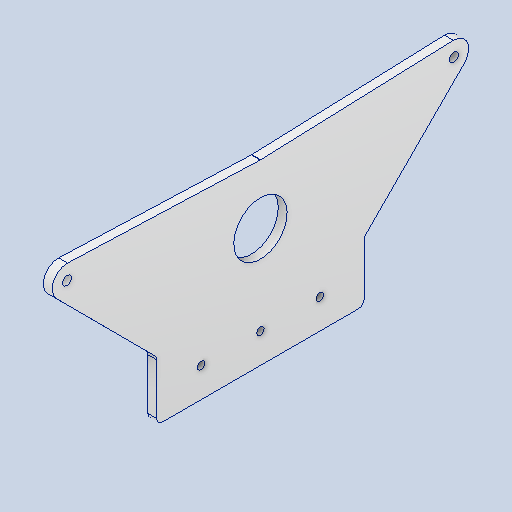
# Autodesk Inventor part: base_weel-v3-Plate-1
Saved by Autodesk Inventor 2025.2 (Build 292293000, 293)
## iProperties
Created: 2025-03-31
Part Number: base_weel-v3-Plate-1
Material: アルミニウム 6061
Document SubType Name: Modeling
Designer: haruy
Density: 2.7 g/cm^3
Appearance: アルミニウム - フラット
Author: haruy
Autodesk Inventor part; units mm, degrees
ref_plane "YZ Plane" through (0, 0, 0) normal (1, 0, 0) x (0, 1, 0)
ref_plane "XZ Plane" through (0, 0, 0) normal (0, 1, 0) x (-1, 0, 0)
ref_plane "XY Plane" through (0, 0, 0) normal (0, 0, 1) x (1, 0, 0)
sketch "スケッチ1" plane through (0, 0, 0) normal (1, 0, 0) x (0, 1, 0)
  line L0 (0, 0) -> (20, 0)
  line L1 (20, 0) -> (20, -110)
  line L2 (20, -110) -> (0, -110)
  line L3 (0, -110) -> (0, 0)
  circle A0 centre (40, -55) radius 52.5
  line L4 (-12.5, 72.5213) -> (-12.5, -343.3137)
  circle A1 centre (40, -55) radius 9.5 construction
  circle A2 centre (40, -55) radius 20
  circle A3 centre (68.2843, -26.7157) radius 20
  circle A4 centre (68.2843, -83.2843) radius 20
  line L5 (68.2843, -26.7157) -> (40, -55)
  line L6 (40, -55) -> (68.2843, -83.2843)
  line L7 (40, -55) -> (40, -2.5)
  line L8 (0, 15) -> (20, 15)
  line L9 (20, 15) -> (20, -125)
  line L10 (20, -125) -> (0, -125)
  line L11 (0, -125) -> (0, 15)
  circle A5 centre (68.2843, -26.7157) radius 23.5
  circle A6 centre (57.4091, 10.2164) radius 5
  circle A7 centre (57.4091, -120.2164) radius 5
  line L12 (20, -20) -> (0, -20)
  line L13 (0, -55) -> (20, -55)
  circle A8 centre (40, -55) radius 9
  circle A9 centre (57.4091, 10.2164) radius 1.5
  circle A10 centre (57.4091, -120.2164) radius 1.5
  line L14 (20, -20) -> (53.8799, 13.7583)
  line L15 (62.4057, 10.0326) -> (59.9865, -55.7352)
  circle A11 centre (10, -55) radius 1.25
  circle A12 centre (10, -35) radius 1.25
  line L16 (20, -90) -> (53.8799, -123.7583)
  line L17 (62.4057, -120.0326) -> (59.9865, -54.2648)
  circle A13 centre (10, -75) radius 1.25
  line L18 (20, -90) -> (0, -90)
  point P0 (0.8688, -20)
  point P1 (0, -20.9963)
  point P2 (0, -89.0037)
  point P3 (0.8688, -90)
  point P4 (60.0135, -55)
  point P5 (0, -90)
  point P6 (0, -20)
  dimension "d2" = 105
  dimension "d6" = 40
  dimension "d0" = 20
  dimension "d1" = 110
  dimension "d3" = 19
  dimension "d4" = 20
  dimension "d5" = 55
  dimension "d7" = 40
  dimension "d8" = 40
  dimension "d9" = 90
  dimension "d10" = 45
  dimension "d11" = 20
  dimension "d12" = 140
  dimension "d13" = 70
  dimension "d14" = 0
  dimension "d15" = 47
  dimension "d16" = 10
  dimension "d17" = 10
  dimension "d18" = 67.5
  dimension "d19" = 67.5
  dimension "d20" = 38.5
  dimension "d21" = 38.5
  dimension "d22" = 20
  dimension "d23" = 18
  dimension "d24" = 3
  dimension "d25" = 3
  dimension "d26" = 2.5
  dimension "d27" = 2.5
  dimension "d28" = 10
  dimension "d29" = 20
  constraints: 38 end point, 12 centre point, 6 coincident, 6 parallel, 5 symmetric about line, 3 midpoint, 3 perpendicular, 3 point on line, 2 horizontal, 2 point on circle, 2 tangent, 2 vertical, 10 other
  measures "d0" distance of L1.end L2.end
  measures "d1" distance of L0.end L1.end
  measures "d3" diameter of A1
  measures "d4" distance from line of L1 point (40, -55)
  measures "d5" distance from line of point (40, -55) L0
  measures "d7" diameter of A3
  measures "d8" diameter of A4
  measures "d11" distance of L9.end L10.end
  measures "d12" distance between parallel lines of L10 L8
  measures "d13" distance from line of L13.start L8
  measures "d14" distance between parallel lines of L3 L11
  measures "d15" diameter of A5
  measures "d16" diameter of A6
  measures "d17" diameter of A7
  measures "d18" distance of A6.centre point (40, -55)
  measures "d19" distance of A7.centre L5.end
  measures "d20" distance of A6.centre L5.start
  measures "d21" distance of A7.centre L6.end
  measures "d22" distance between parallel lines of L0 L12
  measures "d23" diameter of A8
  measures "d24" diameter of A9
  measures "d25" diameter of A10
  measures "d26" diameter of A11
  measures "d27" diameter of A12
  measures "d28" distance from line of A12.centre L3
  measures "d29" distance of A11.centre A12.centre
extrude "押し出し1" add sketch "スケッチ1" against normal blind 3 contours L12 A0 L3 | A0 L12 L1 L13 A11 L3 | L14 A0 L7 A2 L1 | L14 A6 L15 A5 A0 | L13 A11 L1 L18 A0 L3 | A2 A4 L17 A0 L16 L1 | A2 L7 A8 L6 | A0 A5 A2 L7 | A6 | A0 L18 L3 | A2 A5 L5 A8 L7 | L6 A8 L5 A5 A2 | A2 L15 L17 A4 | L6 L17 A4 | A4 L17 L6 | A5 L15 A0 | A0 L15 A3 A2 A5 | A0 L17 A7 L16 | A2 L5 A5 | A2 L17 L15 | A7 | A3 L15 A5 A2 | L5 L15 A3 | A3 L15 L5 | A2 A5 L5 | L17 A2 A5 L15
fillet "フィレット1" radius 2 5 edges at (-1.5, 20, -90) (-1.5, 0, -90) (-1.5, 0, -20) (-1.5, 20, -20) (-1.5, 60.0135, -55)
equation "\"d19\" = d18"
equation "\"d21\" = d20"
